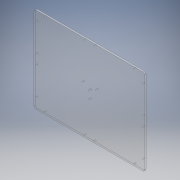
# Autodesk Inventor part: frame_lowerl
Saved by Autodesk Inventor 2017 (Build 210142000, 142)
## iProperties
Created: 2017-04-26
Part Number: frame_lowerl
Material: Tworzywo sztuczne PMMA
Document SubType Name: Modeling
Designer: Speed King
Density: 1.188 g/cm^3
Appearance: Poliwęglan — przezroczysty
Mass: 527.903 g
Surface Area: 1837.12 cm^2
Volume: 444.363 cm^3
Author: Speed King
Autodesk Inventor part; units mm, degrees
ref_plane "YZ Plane" through (0, 0, 0) normal (1, 0, 0) x (0, 1, 0)
ref_plane "XZ Plane" through (0, 0, 0) normal (0, 1, 0) x (-1, 0, 0)
ref_plane "XY Plane" through (0, 0, 0) normal (0, 0, 1) x (1, 0, 0)
sketch "Szkic1" plane through (0, 0, 0) normal (0, 1, 0) x (-1, 0, 0)
  line L0 (-169, -131.5) -> (169, -131.5)
  line L1 (169, -131.5) -> (169, 131.5)
  line L2 (169, 131.5) -> (-169, 131.5)
  line L3 (-169, 131.5) -> (-169, -131.5)
  line L4 (-169, -131.5) -> (169, 131.5) construction
  line L5 (169, -131.5) -> (-169, 131.5) construction
  point P0 (0, 0)
  dimension "d0" = 338
  dimension "d1" = 263
  constraints: 12 end point, 2 midpoint, 2 parallel, 1 horizontal, 1 perpendicular
  measures "d0" distance of L2.end L1.end
  measures "d1" distance of L1.end L0.end
extrude "Wyciągnięcie proste1" add sketch "Szkic1" along normal blind 5
fillet "Zaokrąglenie1" radius 5 4 edges at (-169, 2.5, -131.5) (169, 2.5, -131.5) (-169, 2.5, 131.5) (169, 2.5, 131.5)
sketch "Szkic2" plane through (0, 0, 0) normal (0, -1, 0) x (1, 0, 0)
  circle A0 centre (-137.5, 126.2) radius 1.65 projected
  circle A1 centre (-163.7, 100) radius 1.65 projected
  circle A2 centre (-163.7, 15) radius 1.65 projected
  circle A3 centre (-163.7, -15) radius 1.65 projected
  circle A4 centre (-163.7, -100) radius 1.65 projected
  circle A5 centre (-137.5, -126.2) radius 1.65 projected
  circle A6 centre (-15, -126.2) radius 1.65 projected
  circle A7 centre (15, -126.2) radius 1.65 projected
  circle A8 centre (-20.7846, 12) radius 2.25 projected
  circle A9 centre (0, -24) radius 2.25 projected
  circle A10 centre (20.7846, 12) radius 2.25 projected
  circle A11 centre (137.5, -126.2) radius 1.65 projected
  circle A12 centre (163.7, -100) radius 1.65 projected
  circle A13 centre (163.7, -15) radius 1.65 projected
  circle A14 centre (163.7, 15) radius 1.65 projected
  circle A15 centre (163.7, 100) radius 1.65 projected
  circle A16 centre (137.5, 126.2) radius 1.65 projected
  circle A17 centre (15, 126.2) radius 1.65 projected
  circle A18 centre (-15, 126.2) radius 1.65 projected
  point P0 (0, 0)
hole "Otwór2" at (20.7846, 0, 12) at (-20.7846, 0, 12) at (0, 0, -24) direction (0, 1, 0) diameter 4 end through all
hole "Otwór1" at (137.5, 0, -126.2) at (163.7, 0, -100) at (163.7, 0, -15) at (163.7, 0, 15) at (163.7, 0, 100) at (137.5, 0, 126.2) at (15, 0, 126.2) at (-15, 0, 126.2) at (-137.5, 0, 126.2) at (-163.7, 0, 100) at (-163.7, 0, 15) at (-163.7, 0, -15) at (-163.7, 0, -100) at (-137.5, 0, -126.2) at (-15, 0, -126.2) at (15, 0, -126.2) direction (0, 1, 0) diameter 3 end through all
sketch "Szkic3" plane through (0, 0, 0) normal (0, -1, 0) x (1, 0, 0)
  circle A0 centre (0, 0) radius 2.5
  dimension "d27" = 5
  constraints: 1 centre point, 1 coincident
  measures "d27" diameter of A0
extrude "Wyciągnięcie proste3" cut sketch "Szkic3" against normal through all
